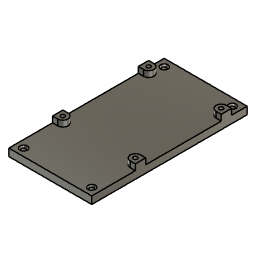
Pi v3 (Autodesk Fusion 360 design; units mm, degrees)
Autodesk Fusion 360 part; units mm, degrees
sketch "Sketch1" plane through (0, 0, 0) normal (0, 0, 1) x (1, 0, 0)
  line L0 (0, 0) -> (56, 0)
  line L1 (56, 0) -> (56, 105)
  line L2 (56, 105) -> (0, 105)
  line L3 (0, 105) -> (0, 0)
  dimension "d1" = 56
  dimension "d2" = 105
  constraint horizontal L0
  constraint vertical L1
  constraint horizontal L2
  constraint vertical L3
  constraint coincident L0.start L3.end
  measures "d1" distance of L0.start L0.end
  measures "d2" distance of L0.start L2.end
extrude "Extrude1" add sketch "Sketch1" along normal blind 5
sketch "Sketch2" plane through (0, 0, 5) normal (0, 0, 1) x (-1, 0, 0)
  line L0 (0, -105) -> (0, 0)
  line L1 (0, 0) -> (-56, 0)
  line L2 (-56, 0) -> (-56, -105)
  line L3 (-56, -105) -> (0, -105)
  circle A0 centre (-3.5, -91) radius 1.35
  circle A1 centre (-52.5, -91) radius 1.35
  circle A2 centre (-3.5, -33) radius 1.35
  circle A3 centre (-52.5, -33) radius 1.35
  circle A4 centre (-3.5, -91) radius 3.5
  circle A5 centre (-52.5, -91) radius 3.5
  circle A6 centre (-52.5, -33) radius 3.5
  circle A7 centre (-3.5, -33) radius 3.5
  line L4 (-3.5, -36.5) -> (0, -36.5)
  line L5 (-3.5, -29.5) -> (0, -29.5)
  line L6 (-52.5, -29.5) -> (-56, -29.5)
  line L7 (-52.5, -87.5) -> (-56, -87.5)
  line L8 (-52.5, -94.5) -> (-56, -94.5)
  line L9 (-3.5, -94.5) -> (0, -94.5)
  line L10 (-3.5, -87.5) -> (0, -87.5)
  line L11 (-52.5, -36.5) -> (-56, -36.5)
  dimension "d5" = 2.7
  dimension "d6" = 58
  dimension "d7" = 49
  dimension "d8" = 3.5
  dimension "d9" = 56
  dimension "d10" = 105
  dimension "d11" = 33
  constraint vertical A0.centre A2.centre
  constraint horizontal A0.centre A1.centre
  constraint horizontal A2.centre A3.centre
  constraint equal A0 A1
  constraint equal A0 A2
  constraint equal A0 A3
  constraint vertical A1.centre A3.centre
  constraint concentric A0 A4
  constraint concentric A1 A5
  constraint concentric A3 A6
  constraint concentric A2 A7
  constraint tangent L0 A4
  constraint tangent L2 A5
  constraint tangent L2 A6
  constraint tangent L0 A7
  constraint coincident A7 L4.start
  constraint coincident L0 L4.end
  constraint perpendicular L0 L4
  constraint coincident A7 L5.start
  constraint coincident L0 L5.end
  constraint perpendicular L0 L5
  constraint coincident A6 L6.start
  constraint coincident L2 L6.end
  constraint perpendicular L2 L6
  constraint coincident A5 L7.start
  constraint coincident L2 L7.end
  constraint perpendicular L2 L7
  constraint coincident A5 L8.start
  constraint coincident L2 L8.end
  constraint perpendicular L2 L8
  constraint coincident A4 L9.start
  constraint coincident L0 L9.end
  constraint perpendicular L0 L9
  constraint coincident A4 L10.start
  constraint coincident L0 L10.end
  constraint perpendicular L0 L10
  constraint tangent A4 L9
  constraint tangent A4 L10
  constraint tangent A5 L8
  constraint tangent A5 L7
  constraint tangent A6 L6
  constraint tangent A7 L5
  constraint tangent A7 L4
  constraint coincident A6 L11.start
  constraint coincident L2 L11.end
  constraint perpendicular L2 L11
  constraint tangent A6 L11
  measures "d5" diameter of A0
  measures "d6" distance of A0.centre A2.centre
  measures "d7" distance of A2.centre A3.centre
  measures "d8" horizontal distance of L0.end A2.centre
  measures "d9" distance of L0.end L1.end
  measures "d10" distance of L0.start L0.end
  measures "d11" vertical distance of L0.end A2.centre
extrude "Extrude2" add sketch "Sketch2" along normal blind 4 contours L0 A4 L9 | L0 A4 L10 | A4 | L2 A5 L8 | L2 A5 L7 | A5 | L0 A7 L4 | L0 A7 L5 | A7 | L2 A6 L11 | L2 A6 L6 | A6
extrude "Extrude3" cut sketch "Sketch2" against normal blind 7 contours A0 | A1 | A2 | A3
sketch "Sketch3" plane through (0, 0, 5) normal (0, 0, 1) x (-1, 0, 0)
  line L0 (-3.5, -29.5) -> (0, -29.5)
  line L1 (0, -29.5) -> (0, 0)
  line L2 (0, 0) -> (-56, 0)
  line L3 (-56, 0) -> (-56, -29.5)
  line L4 (-56, -29.5) -> (-52.5, -29.5)
  arc A0 (-52.5, -36.5) -> (-52.5, -29.5) centre (-52.5, -33) ccw
  line L5 (-52.5, -36.5) -> (-56, -36.5)
  line L6 (-56, -36.5) -> (-56, -87.5)
  line L7 (-56, -87.5) -> (-52.5, -87.5)
  arc A1 (-52.5, -94.5) -> (-52.5, -87.5) centre (-52.5, -91) ccw
  line L8 (-52.5, -94.5) -> (-56, -94.5)
  line L9 (-56, -94.5) -> (-56, -105)
  line L10 (-56, -105) -> (0, -105)
  line L11 (0, -105) -> (0, -94.5)
  line L12 (0, -94.5) -> (-3.5, -94.5)
  arc A2 (-3.5, -87.5) -> (-3.5, -94.5) centre (-3.5, -91) ccw
  line L13 (-3.5, -87.5) -> (0, -87.5)
  line L14 (0, -87.5) -> (0, -36.5)
  line L15 (0, -36.5) -> (-3.5, -36.5)
  arc A3 (-3.5, -29.5) -> (-3.5, -36.5) centre (-3.5, -33) ccw
  circle A4 centre (-5, -5) radius 1.5
  circle A5 centre (-51, -5) radius 1.5
  circle A6 centre (-51, -100) radius 1.5
  circle A7 centre (-5, -100) radius 1.5
  dimension "d16" = 5
  dimension "d17" = 5
  dimension "d18" = 5
  dimension "d19" = 3
  dimension "d20" = 5
  constraint equal A6 A7
  constraint equal A4 A7
  constraint equal A5 A7
  constraint horizontal A6.centre A7.centre
  constraint vertical A4.centre A7.centre
  constraint horizontal A4.centre A5.centre
  constraint vertical A5.centre A6.centre
  measures "d16" horizontal distance of L10.end A7.centre
  measures "d17" vertical distance of L10.end A7.centre
  measures "d18" horizontal distance of L9.end A6.centre
  measures "d19" diameter of A7
  measures "d20" vertical distance of L1.end A4.centre
extrude "Extrude4" cut sketch "Sketch3" against normal blind 5 contours A4 | A5 | A6 | A7
chamfer "Chamfer1" distance 1 distance2 1 4 edges at (6.3985, 4.4576, 5) (52.3985, 4.4576, 5) (52.3985, 99.4576, 5) (6.3985, 99.4576, 5) measured on face at (35.3731, 53.1886, 5) measured on face at (35.3731, 53.1886, 5) measured on face at (35.3731, 53.1886, 5) measured on face at (35.3731, 53.1886, 5)
sketch "Sketch4" plane through (0, 0, 0) normal (0, 0, -1) x (1, 0, 0)
  circle A0 centre (51, -100) radius 1.5
  circle A1 centre (5, -5) radius 1.5
  circle A2 centre (5, -100) radius 1.5
  circle A3 centre (51, -5) radius 1.5
  circle A4 centre (3.5, -91) radius 1.35
  circle A5 centre (52.5, -91) radius 1.35
  circle A6 centre (3.5, -33) radius 1.35
  circle A7 centre (52.5, -33) radius 1.35
  line L0 (0, 0) -> (0, -105)
  line L1 (0, -105) -> (56, -105)
  line L2 (56, -105) -> (56, 0)
  line L3 (56, 0) -> (0, 0)
  circle A8 centre (3.5, -91) radius 2
  circle A9 centre (52.5, -91) radius 2
  circle A10 centre (52.5, -33) radius 2
  circle A11 centre (3.5, -33) radius 2
  dimension "d25" = 4
  constraint concentric A4 A8
  constraint concentric A5 A9
  constraint concentric A7 A10
  constraint concentric A6 A11
  constraint equal A8 A11
  constraint equal A10 A11
  constraint equal A9 A11
  measures "d25" diameter of A11
extrude "Extrude5" cut sketch "Sketch4" against normal blind 5 contours A8 | A9 | A10 | A11
equation "d2 = 85 mm + 20 mm"
equation "d8 = ( d9 - d7 ) / 2"
equation "d11 = 23 mm + 10 mm"
equation "d17 = d16"
equation "d18 = d16"
